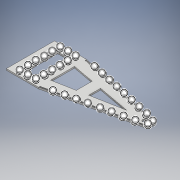
# Autodesk Inventor part: W1suppoert2
Saved by Autodesk Inventor 2017 (Build 210142000, 142)
## iProperties
Created: 2016-12-01
Part Number: W1suppoert2
Material: Generic
Document SubType Name: Sheet Metal
Designer: aesen
Density: 1 g/cm^3
Sheet Metal Rule: Default_mm
Appearance: Default
Author: aesen
Autodesk Inventor part; units mm, degrees
note: some values were not read from the file. Chosen so that the rebuilt part matches the saved one: direction of "Emboss8".
ref_plane "YZ Plane" through (0, 0, 0) normal (1, 0, 0) x (0, 1, 0)
ref_plane "XZ Plane" through (0, 0, 0) normal (0, 1, 0) x (-1, 0, 0)
ref_plane "XY Plane" through (0, 0, 0) normal (0, 0, 1) x (1, 0, 0)
sketch "Sketch1" plane through (0, 0, 0) normal (0, 0, 1) x (1, 0, 0)
  line L0 (-400, 150) -> (-400, 0)
  circle A0 centre (-350, 125) radius 3.5
  circle A1 centre (-300, 125) radius 3.5
  circle A2 centre (-250, 125) radius 3.5
  circle A3 centre (-350, 75) radius 3.5
  circle A4 centre (-250, 75) radius 3.5
  circle A5 centre (-350, 25) radius 3.5
  circle A6 centre (-250, 25) radius 3.5
  line L1 (-330, 100) -> (-270, 100)
  line L2 (-270, 100) -> (-270, 0)
  line L3 (-330, 0) -> (-330, 100)
  line L4 (-400, -150.0109) -> (-400, 0)
  circle A7 centre (-350, -125) radius 3.5
  circle A8 centre (-300, -125) radius 3.5
  circle A9 centre (-250, -125) radius 3.5
  circle A10 centre (-350, -75) radius 3.5
  circle A11 centre (-250, -75) radius 3.5
  circle A12 centre (-350, -25) radius 3.5
  circle A13 centre (-250, -25) radius 3.5
  line L5 (-330, -100) -> (-270, -100)
  line L6 (-270, -100) -> (-270, 0)
  line L7 (-330, 0) -> (-330, -100)
  line L8 (334.439, -20.7765) -> (-199.5823, -140.5264)
  line L9 (-199.5608, -75) -> (200.433, 0.033)
  line L10 (340.7459, -25.7251) -> (-199.5823, -146.9202)
  line L11 (-199.5588, -150.0109) -> (343.8125, -28.1391)
  line L12 (-400, -150.0109) -> (-199.5588, -150.0109)
  circle A14 centre (-139.6396, -130.2873) radius 3.5
  circle A15 centre (-79.6396, -116.8294) radius 3.5
  circle A16 centre (-19.6396, -103.3714) radius 3.5
  circle A17 centre (40.3604, -89.9135) radius 3.5
  circle A18 centre (100.3828, -76.4523) radius 3.5
  circle A19 centre (160.3828, -62.9943) radius 3.5
  circle A20 centre (220.3828, -49.5364) radius 3.5
  circle A21 centre (280.3828, -36.0784) radius 3.5
  line L13 (334.439, -20.7765) -> (334.4401, -0.0632)
  circle A22 centre (337.6443, -15.0341) radius 3.5
  line L14 (340.7459, -25.7251) -> (340.7459, -0.0341)
  line L15 (343.8125, -28.1391) -> (343.8125, -0.0055)
  line L16 (334.4412, 20.65) -> (-199.567, 140.4581)
  line L17 (-199.5608, 74.9977) -> (200.433, 0.033)
  line L18 (340.7612, 25.6568) -> (-199.567, 146.8519)
  line L19 (-199.5588, 150) -> (343.8125, 28.1281)
  line L20 (-400, 150) -> (-199.5588, 150)
  circle A23 centre (-139.6172, 130.2158) radius 3.5
  circle A24 centre (-79.6172, 116.7578) radius 3.5
  circle A25 centre (-19.6172, 103.2999) radius 3.5
  circle A26 centre (40.3828, 89.8419) radius 3.5
  circle A27 centre (100.3828, 76.384) radius 3.5
  circle A28 centre (160.3828, 62.926) radius 3.5
  circle A29 centre (220.3828, 49.4681) radius 3.5
  circle A30 centre (280.3828, 36.0102) radius 3.5
  line L21 (334.4412, 20.65) -> (334.4401, -0.0632)
  circle A31 centre (337.6443, 14.9659) radius 3.5
  line L22 (340.7612, 25.6568) -> (340.7459, -0.0341)
  line L23 (343.8125, 28.1281) -> (343.8125, -0.0055)
  line L24 (0.4361, -37.4835) -> (0.4361, 37.5153)
  line L25 (-63.8167, -49.5364) -> (-63.8167, 49.5572)
  line L26 (-199.5823, -146.9202) -> (-199.5823, -140.5264)
  line L27 (-199.5608, -75) -> (-199.5608, 74.9977)
  line L28 (-199.567, 140.4581) -> (-199.567, 146.8519)
  circle A32 centre (313.3483, 0) radius 12.7
  point P0 (0, 0)
  dimension "d182" = 25.4
  constraints: 58 end point, 33 centre point, 4 vertical, 2 horizontal, 2 midpoint, 2 point on line, 1 parallel, 1 perpendicular
  measures "d182" diameter of A32
sketch "Sketch9" plane through (0, 0, 0) normal (0, 0, 1) x (1, 0, 0)
  line L0 (-400, 150) -> (-400, 0)
  circle A0 centre (-350, 125) radius 3.5
  circle A1 centre (-300, 125) radius 3.5
  circle A2 centre (-250, 125) radius 3.5
  circle A3 centre (-350, 75) radius 3.5
  circle A4 centre (-250, 75) radius 3.5
  circle A5 centre (-350, 25) radius 3.5
  circle A6 centre (-250, 25) radius 3.5
  line L1 (-330, 100) -> (-270, 100)
  line L2 (-270, 100) -> (-270, 0)
  line L3 (-330, 0) -> (-330, 100)
  line L4 (334.439, -20.7765) -> (-199.5823, -140.5264)
  line L5 (-199.5608, -75) -> (200.433, 0.033)
  circle A7 centre (-300, -125) radius 3.5
  circle A8 centre (-250, -125) radius 3.5
  circle A9 centre (-350, -125) radius 3.5
  circle A10 centre (-250, -25) radius 3.5
  line L6 (-270, -100) -> (-270, 0)
  circle A11 centre (-350, -25) radius 3.5
  line L7 (-330, -100) -> (-270, -100)
  circle A12 centre (-350, -75) radius 3.5
  line L8 (-330, 0) -> (-330, -100)
  line L9 (-400, -150.0109) -> (-400, 0)
  circle A13 centre (-250, -75) radius 3.5
  line L10 (340.7459, -25.7251) -> (-199.5823, -146.9202)
  line L11 (-199.5588, -150.0109) -> (343.8125, -28.1391)
  line L12 (-400, -150.0109) -> (-199.5588, -150.0109)
  circle A14 centre (-139.6396, -130.2873) radius 3.5
  circle A15 centre (-79.6396, -116.8294) radius 3.5
  circle A16 centre (-19.6396, -103.3714) radius 3.5
  circle A17 centre (40.3604, -89.9135) radius 3.5
  circle A18 centre (100.3828, -76.4523) radius 3.5
  circle A19 centre (160.3828, -62.9943) radius 3.5
  circle A20 centre (220.3828, -49.5364) radius 3.5
  circle A21 centre (280.3828, -36.0784) radius 3.5
  line L13 (334.439, -20.7765) -> (334.4401, -0.0632)
  circle A22 centre (337.6443, -15.0341) radius 3.5
  line L14 (340.7459, -25.7251) -> (340.7459, -0.0341)
  line L15 (343.8125, -28.1391) -> (343.8125, -0.0055)
  line L16 (-400, 150) -> (-199.5588, 150)
  circle A23 centre (160.3828, 62.926) radius 3.5
  circle A24 centre (100.3828, 76.384) radius 3.5
  circle A25 centre (40.3828, 89.8419) radius 3.5
  circle A26 centre (-19.6172, 103.2999) radius 3.5
  line L17 (-199.5608, 74.9977) -> (200.433, 0.033)
  line L18 (334.4412, 20.65) -> (-199.567, 140.4581)
  line L19 (-199.5588, 150) -> (343.8125, 28.1281)
  line L20 (340.7612, 25.6568) -> (-199.567, 146.8519)
  line L21 (343.8125, 28.1281) -> (343.8125, -0.0055)
  circle A27 centre (220.3828, 49.4681) radius 3.5
  circle A28 centre (280.3828, 36.0102) radius 3.5
  line L22 (334.4412, 20.65) -> (334.4401, -0.0632)
  circle A29 centre (337.6443, 14.9659) radius 3.5
  line L23 (340.7612, 25.6568) -> (340.7459, -0.0341)
  circle A30 centre (-139.6172, 130.2158) radius 3.5
  circle A31 centre (-79.6172, 116.7578) radius 3.5
  line L24 (0.4361, -37.4835) -> (0.4361, 37.5153)
  line L25 (-63.8167, -49.5364) -> (-63.8167, 49.5572)
  line L26 (-199.5823, -146.9202) -> (-199.5823, -140.5264)
  line L27 (-199.5608, -75) -> (-199.5608, 74.9977)
  line L28 (-199.567, 140.4581) -> (-199.567, 146.8519)
  circle A32 centre (313.3483, 0) radius 12.7
  point P0 (0, 0)
  point P1 (0, 0)
  dimension "d273" = 25.4
  constraints: 58 end point, 33 centre point, 4 vertical, 2 horizontal, 2 midpoint, 2 point on line, 1 parallel, 1 perpendicular
  measures "d273" diameter of A32
sketch "Sketch11" plane through (0, 0, 0) normal (0, 0, 1) x (1, 0, 0)
  line L0 (-400, 150) -> (-400, 0)
  circle A0 centre (-350, 125) radius 3.5
  circle A1 centre (-300, 125) radius 3.5
  circle A2 centre (-250, 125) radius 3.5
  circle A3 centre (-350, 75) radius 3.5
  circle A4 centre (-250, 75) radius 3.5
  circle A5 centre (-350, 25) radius 3.5
  circle A6 centre (-250, 25) radius 3.5
  line L1 (-330, 100) -> (-270, 100)
  line L2 (-270, 100) -> (-270, 0)
  line L3 (-330, 0) -> (-330, 100)
  line L4 (334.439, -20.7765) -> (-199.5823, -140.5264)
  line L5 (-199.5608, -75) -> (200.433, 0.033)
  circle A7 centre (-300, -125) radius 3.5
  circle A8 centre (-250, -125) radius 3.5
  circle A9 centre (-350, -125) radius 3.5
  circle A10 centre (-250, -25) radius 3.5
  line L6 (-270, -100) -> (-270, 0)
  circle A11 centre (-350, -25) radius 3.5
  line L7 (-330, -100) -> (-270, -100)
  circle A12 centre (-350, -75) radius 3.5
  line L8 (-330, 0) -> (-330, -100)
  line L9 (-400, -150.0109) -> (-400, 0)
  circle A13 centre (-250, -75) radius 3.5
  line L10 (340.7459, -25.7251) -> (-199.5823, -146.9202)
  line L11 (-199.5588, -150.0109) -> (343.8125, -28.1391)
  line L12 (-400, -150.0109) -> (-199.5588, -150.0109)
  circle A14 centre (-139.6396, -130.2873) radius 3.5
  circle A15 centre (-79.6396, -116.8294) radius 3.5
  circle A16 centre (-19.6396, -103.3714) radius 3.5
  circle A17 centre (40.3604, -89.9135) radius 3.5
  circle A18 centre (100.3828, -76.4523) radius 3.5
  circle A19 centre (160.3828, -62.9943) radius 3.5
  circle A20 centre (220.3828, -49.5364) radius 3.5
  circle A21 centre (280.3828, -36.0784) radius 3.5
  line L13 (334.439, -20.7765) -> (334.4401, -0.0632)
  circle A22 centre (337.6443, -15.0341) radius 3.5
  line L14 (340.7459, -25.7251) -> (340.7459, -0.0341)
  line L15 (343.8125, -28.1391) -> (343.8125, -0.0055)
  line L16 (-400, 150) -> (-199.5588, 150)
  circle A23 centre (160.3828, 62.926) radius 3.5
  circle A24 centre (100.3828, 76.384) radius 3.5
  circle A25 centre (40.3828, 89.8419) radius 3.5
  circle A26 centre (-19.6172, 103.2999) radius 3.5
  line L17 (-199.5608, 74.9977) -> (200.433, 0.033)
  line L18 (334.4412, 20.65) -> (-199.567, 140.4581)
  line L19 (-199.5588, 150) -> (343.8125, 28.1281)
  line L20 (340.7612, 25.6568) -> (-199.567, 146.8519)
  line L21 (343.8125, 28.1281) -> (343.8125, -0.0055)
  circle A27 centre (220.3828, 49.4681) radius 3.5
  circle A28 centre (280.3828, 36.0102) radius 3.5
  line L22 (334.4412, 20.65) -> (334.4401, -0.0632)
  circle A29 centre (337.6443, 14.9659) radius 3.5
  line L23 (340.7612, 25.6568) -> (340.7459, -0.0341)
  circle A30 centre (-139.6172, 130.2158) radius 3.5
  circle A31 centre (-79.6172, 116.7578) radius 3.5
  line L24 (0.4361, -37.4835) -> (0.4361, 37.5153)
  line L25 (-63.8167, -49.5364) -> (-63.8167, 49.5572)
  line L26 (-199.5823, -146.9202) -> (-199.5823, -140.5264)
  line L27 (-199.5608, -75) -> (-199.5608, 74.9977)
  line L28 (-199.567, 140.4581) -> (-199.567, 146.8519)
  circle A32 centre (313.3483, 0) radius 12.7
  point P0 (0, 0)
  point P1 (0, 0)
  dimension "d275" = 25.4
  constraints: 58 end point, 33 centre point, 4 vertical, 2 horizontal, 2 midpoint, 2 point on line, 1 parallel, 1 perpendicular
  measures "d275" diameter of A32
extrude "Extrusion10" add sketch "Sketch9" against normal blind 9.525 contours L16 L19 L21 L15 L11 L12 L9 L0 | A0 | A1 | A2 | A3 | A4 | A5 | A6 | L13 A22 L14 L10 A21 L4 | A21 L10 L4 | L4 A21 | A22 L13 | L13 A22 L14 | A21 L10 A20 L4 | L13 L22 A29 L23 L14 A22 | L14 A22 | A20 L10 L4 | L4 A20 | L10 A21 | A20 L10 A19 L4 | A20 L10 | A29 L22 | L22 A29 L23 | A19 L10 L4 | L4 A19 | L22 L18 A28 L20 L23 A29 | L23 A29 | A19 L10 A18 L4 | A19 L10 | A18 L10 L4 | L4 A18 | A28 L18 | L18 A28 L20 | A18 L10 A17 L4 | A18 L10 | L18 A27 L20 A28 | L20 A28 | A17 L10 L4 | L4 A17 | A27 L18 | L18 A27 L20 | A17 L10 A16 L4 | A17 L10 | L18 A23 L20 A27 | L20 A27 | A16 L10 L4 | L4 A16 | L18 A23 L20 | A23 L18 | A16 L10 A15 L4 | A16 L10 | L18 A24 L20 A23 | L20 A23 | A15 L10 L4 | L4 A15 | L18 A24 L20 | A24 L18 | A15 L10 A14 L4 | A15 L10 | L20 A24 | L18 A25 L20 A24 | A14 L10 L4 | L4 A14 | L18 A25 L20 | A25 L18 | A14 L10 L26 L4 | A14 L10 | L20 A25 | L18 A26 L20 A25 | L18 A26 L20 | A26 L18 | L20 A26 | L18 A31 L20 A26 | A31 L18 | L18 A31 L20 | L20 A31 | L18 A30 L20 A31 | A30 L18 | L18 A30 L20 | L20 A30 | L18 L28 L20 A30 | L25 L17 L24 L5 | A7 | A8 | A9 | A10 | A11 | A12 | A13
emboss "Emboss8" sketch "Sketch9" operation cut depth 3 direction (0, 0, -1) contours L13 A22 L14 L10 A21 L4 | A21 L10 L4 | L13 A22 L14 | A21 L10 A20 L4 | L13 L22 A29 L23 L14 A22 | A20 L10 L4 | A20 L10 A19 L4 | L22 A29 L23 | A19 L10 L4 | L22 L18 A28 L20 L23 A29 | A19 L10 A18 L4 | A18 L10 L4 | L18 A28 L20 | A18 L10 A17 L4 | L18 A27 L20 A28 | A17 L10 L4 | L18 A27 L20 | A17 L10 A16 L4 | L18 A23 L20 A27 | A16 L10 L4 | L18 A23 L20 | A16 L10 A15 L4 | L18 A24 L20 A23 | A15 L10 L4 | L18 A24 L20 | A15 L10 A14 L4 | L18 A25 L20 A24 | A14 L10 L4 | L18 A25 L20 | A14 L10 L26 L4 | L18 A26 L20 A25 | L18 A26 L20 | L18 A31 L20 A26 | L18 A31 L20 | L18 A30 L20 A31 | L18 A30 L20 | L18 L28 L20 A30
sketch "Sketch10" plane through (0, 0, 0) normal (0, 0, 1) x (1, 0, 0)
  line L0 (-400, 150) -> (-400, 0)
  circle A0 centre (-350, 125) radius 3.5
  circle A1 centre (-300, 125) radius 3.5
  circle A2 centre (-250, 125) radius 3.5
  circle A3 centre (-350, 75) radius 3.5
  circle A4 centre (-250, 75) radius 3.5
  circle A5 centre (-350, 25) radius 3.5
  circle A6 centre (-250, 25) radius 3.5
  line L1 (-330, 100) -> (-270, 100)
  line L2 (-270, 100) -> (-270, 0)
  line L3 (-330, 0) -> (-330, 100)
  line L4 (334.439, -20.7765) -> (-199.5823, -140.5264)
  line L5 (-199.5608, -75) -> (200.433, 0.033)
  circle A7 centre (-300, -125) radius 3.5
  circle A8 centre (-250, -125) radius 3.5
  circle A9 centre (-350, -125) radius 3.5
  circle A10 centre (-250, -25) radius 3.5
  line L6 (-270, -100) -> (-270, 0)
  circle A11 centre (-350, -25) radius 3.5
  line L7 (-330, -100) -> (-270, -100)
  circle A12 centre (-350, -75) radius 3.5
  line L8 (-330, 0) -> (-330, -100)
  line L9 (-400, -150.0109) -> (-400, 0)
  circle A13 centre (-250, -75) radius 3.5
  line L10 (340.7459, -25.7251) -> (-199.5823, -146.9202)
  line L11 (-199.5588, -150.0109) -> (343.8125, -28.1391)
  line L12 (-400, -150.0109) -> (-199.5588, -150.0109)
  circle A14 centre (-139.6396, -130.2873) radius 3.5
  circle A15 centre (-79.6396, -116.8294) radius 3.5
  circle A16 centre (-19.6396, -103.3714) radius 3.5
  circle A17 centre (40.3604, -89.9135) radius 3.5
  circle A18 centre (100.3828, -76.4523) radius 3.5
  circle A19 centre (160.3828, -62.9943) radius 3.5
  circle A20 centre (220.3828, -49.5364) radius 3.5
  circle A21 centre (280.3828, -36.0784) radius 3.5
  line L13 (334.439, -20.7765) -> (334.4401, -0.0632)
  circle A22 centre (337.6443, -15.0341) radius 3.5
  line L14 (340.7459, -25.7251) -> (340.7459, -0.0341)
  line L15 (343.8125, -28.1391) -> (343.8125, -0.0055)
  line L16 (-400, 150) -> (-199.5588, 150)
  circle A23 centre (160.3828, 62.926) radius 3.5
  circle A24 centre (100.3828, 76.384) radius 3.5
  circle A25 centre (40.3828, 89.8419) radius 3.5
  circle A26 centre (-19.6172, 103.2999) radius 3.5
  line L17 (-199.5608, 74.9977) -> (200.433, 0.033)
  line L18 (334.4412, 20.65) -> (-199.567, 140.4581)
  line L19 (-199.5588, 150) -> (343.8125, 28.1281)
  line L20 (340.7612, 25.6568) -> (-199.567, 146.8519)
  line L21 (343.8125, 28.1281) -> (343.8125, -0.0055)
  circle A27 centre (220.3828, 49.4681) radius 3.5
  circle A28 centre (280.3828, 36.0102) radius 3.5
  line L22 (334.4412, 20.65) -> (334.4401, -0.0632)
  circle A29 centre (337.6443, 14.9659) radius 3.5
  line L23 (340.7612, 25.6568) -> (340.7459, -0.0341)
  circle A30 centre (-139.6172, 130.2158) radius 3.5
  circle A31 centre (-79.6172, 116.7578) radius 3.5
  line L24 (0.4361, -37.4835) -> (0.4361, 37.5153)
  line L25 (-63.8167, -49.5364) -> (-63.8167, 49.5572)
  line L26 (-199.5823, -146.9202) -> (-199.5823, -140.5264)
  line L27 (-199.5608, -75) -> (-199.5608, 74.9977)
  line L28 (-199.567, 140.4581) -> (-199.567, 146.8519)
  circle A32 centre (313.3483, 0) radius 12.7
  point P0 (0, 0)
  point P1 (0, 0)
  dimension "d274" = 25.4
  constraints: 58 end point, 33 centre point, 4 vertical, 2 horizontal, 2 midpoint, 2 point on line, 1 parallel, 1 perpendicular
  measures "d274" diameter of A32
sketch "Sketch15" plane through (0, 0, -9.525) normal (0, 0, -1) x (-1, 0, 0)
  circle A0 centre (350, -125) radius 3.5
  circle A1 centre (300, -125) radius 3.5
  circle A2 centre (250, -125) radius 3.5
  circle A3 centre (350, -75) radius 3.5
  circle A4 centre (250, -75) radius 3.5
  circle A5 centre (350, -25) radius 3.5
  circle A6 centre (250, -25) radius 3.5
  circle A7 centre (139.6172, -130.2158) radius 3.5
  circle A8 centre (139.6396, 130.2873) radius 3.5
  circle A9 centre (79.6396, 116.8294) radius 3.5
  circle A10 centre (19.6396, 103.3714) radius 3.5
  circle A11 centre (79.6172, -116.7578) radius 3.5
  circle A12 centre (19.6172, -103.2999) radius 3.5
  circle A13 centre (-40.3604, 89.9135) radius 3.5
  circle A14 centre (-40.3828, -89.8419) radius 3.5
  circle A15 centre (-100.3828, -76.384) radius 3.5
  circle A16 centre (-160.3828, 62.9943) radius 3.5
  circle A17 centre (-160.3828, -62.926) radius 3.5
  circle A18 centre (-220.3828, 49.5364) radius 3.5
  circle A19 centre (-220.3828, -49.4681) radius 3.5
  circle A20 centre (-100.3828, 76.4523) radius 3.5
  circle A21 centre (-337.6443, 15.0341) radius 3.5
  circle A22 centre (-280.3828, 36.0784) radius 3.5
  circle A23 centre (350, 25) radius 3.5
  circle A24 centre (250, 25) radius 3.5
  circle A25 centre (350, 75) radius 3.5
  circle A26 centre (250, 75) radius 3.5
  circle A27 centre (250, 125) radius 3.5
  circle A28 centre (300, 125) radius 3.5
  circle A29 centre (350, 125) radius 3.5
  circle A30 centre (-280.3828, -36.0102) radius 3.5
  circle A31 centre (-337.6443, -14.9659) radius 3.5
  constraints: 32 centre point
hole "Hole13" at (-350, -125, -9.525) at (-300, -125, -9.525) at (-250, -125, -9.525) at (-350, -75, -9.525) at (-250, -75, -9.525) at (-350, -25, -9.525) at (-250, -25, -9.525) at (-139.6172, -130.2158, -9.525) at (-139.6396, 130.2873, -9.525) at (-250, 25, -9.525) at (-250, 75, -9.525) at (-250, 125, -9.525) at (-300, 125, -9.525) at (-350, 75, -9.525) at (-350, 125, -9.525) at (-350, 25, -9.525) at (-79.6172, -116.7578, -9.525) at (-79.6396, 116.8294, -9.525) at (-19.6396, 103.3714, -9.525) at (-19.6172, -103.2999, -9.525) at (40.3604, 89.9135, -9.525) at (40.3828, -89.8419, -9.525) at (100.3828, 76.4523, -9.525) at (160.3828, 62.9943, -9.525) at (160.3828, -62.926, -9.525) at (220.3828, 49.5364, -9.525) at (220.3828, -49.4681, -9.525) at (280.3828, 36.0784, -9.525) at (280.3828, -36.0102, -9.525) at (337.6443, 15.0341, -9.525) at (337.6443, -14.9659, -9.525) at (100.3828, -76.384, -9.525) direction (0, 0, 1) diameter 3 depth 19.05 tip angle 118 countersink diameter 7 countersink angle 90
equation "\"GapSize\" = Thickness"
equation "\"BendRadius\" = Thickness"
equation "\"BendReliefWidth\" = Thickness"
equation "\"BendReliefDepth\" = 0.5 * Thickness"
equation "\"CornerReliefSize\" = 4 * Thickness"
equation "\"MinimumRemnant\" = 2 * Thickness"
equation "\"TransitionRadius\" = BendRadius"
equation "\"JacobiRadiusSize\" = BendRadius"
equation "\"Thickness\" = 0.5"
body "Solid9"
